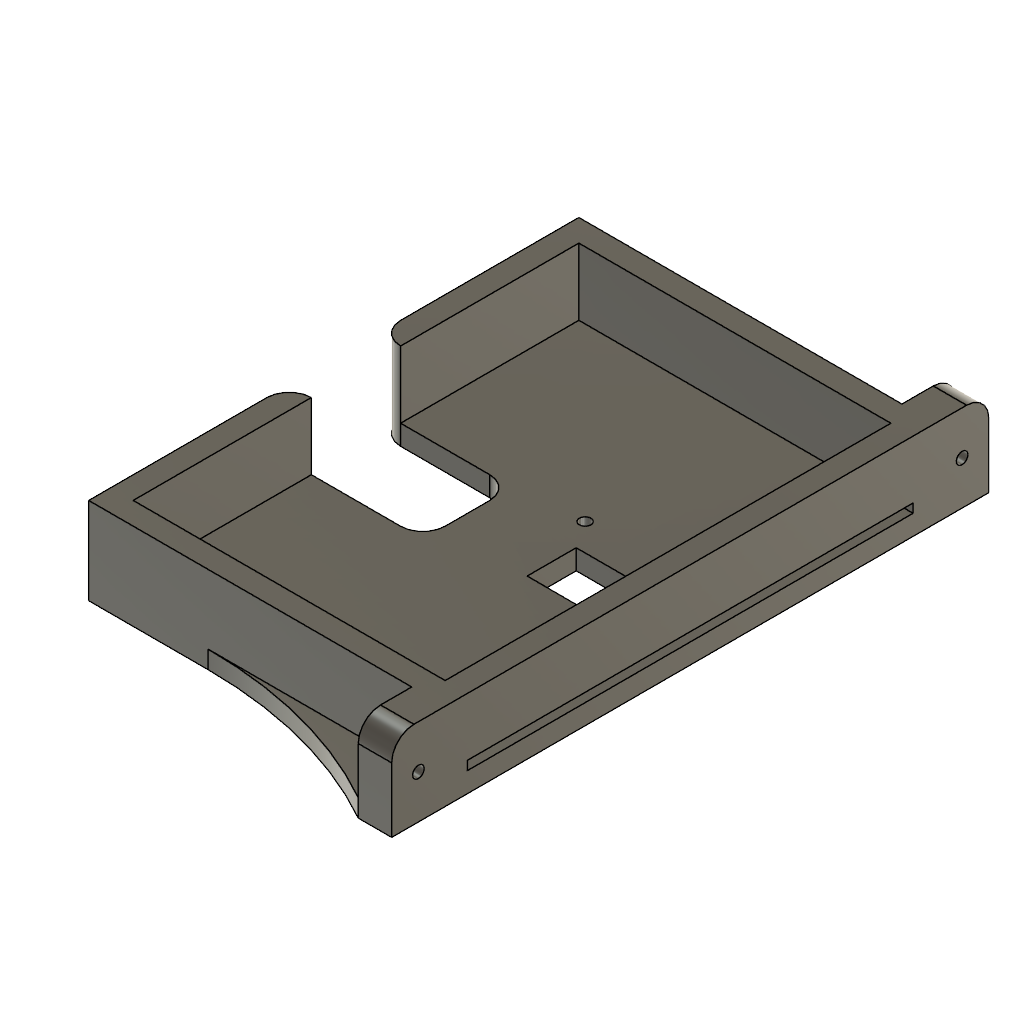
Upper_Card_Holder (Autodesk Fusion 360 design; units mm, degrees)
Autodesk Fusion 360 part; units mm, degrees
sketch "Çizim1" plane through (0, 0, 0) normal (0, 0, 1) x (1, 0, 0)
  line L0 (35, 50) -> (-35, 50)
  line L1 (-35, 50) -> (-35, -50)
  line L2 (-35, -50) -> (35, -50)
  line L3 (35, -50) -> (35, 50)
  line L4 (35, 50) -> (-35, -50) construction
  line L5 (-35, 50) -> (35, -50) construction
  line L6 (-40, -55) -> (40, -55)
  line L7 (40, -55) -> (40, 55)
  line L8 (40, 55) -> (-40, 55)
  line L9 (-40, 55) -> (-40, -55)
  dimension "d1" = 70
  dimension "d2" = 100
  dimension "d3" = 5
  constraint horizontal L0
  constraint perpendicular L0 L1
  constraint parallel L0 L2
  constraint parallel L1 L3
  constraint coincident L4 origin
  constraint coincident L5 origin
  measures "d1" distance of L1.end L2.end
  measures "d2" distance of L0.end L1.end
extrude "Ekstrüzyon1" add sketch "Çizim1" against normal blind 5 contours L0 L1 L2 L3 | L6 L7 L8 L9
extrude "Ekstrüzyon2" add sketch "Çizim1" along normal blind 20
sketch "Çizim2" plane through (0, -50, 0) normal (0, 1, 0) x (-1, 0, 0)
  line L0 (-35, 0) -> (35, 0)
  line L1 (35, 0) -> (35, 20)
  line L2 (35, 20) -> (-35, 20)
  line L3 (-35, 20) -> (-35, 0)
  line L4 (-35, 0) -> (35, 0)
  line L5 (35, 0) -> (35, 2.4)
  line L6 (35, 2.4) -> (-35, 2.4)
  line L7 (-35, 2.4) -> (-35, 0)
  dimension "d8" = 2.4
  constraint horizontal L4
  constraint vertical L5
  constraint horizontal L6
  constraint vertical L7
  constraint coincident L0.start L3.end
  measures "d8" distance of L0.start L6.end
sketch "Çizim3" plane through (0, 0, 20) normal (0, 0, 1) x (-1, 0, 0)
  line L0 (-35, -50) -> (-35, 50)
  line L1 (-35, 50) -> (35, 50)
  line L2 (35, 50) -> (35, -50)
  line L3 (35, -50) -> (-35, -50)
  line L4 (40, -55) -> (40, 55)
  line L5 (40, 55) -> (-40, 55)
  line L6 (-40, 55) -> (-40, -55)
  line L7 (-40, -55) -> (40, -55)
  line L8 (12, -12.5) -> (-12, -12.5)
  line L9 (-12, -12.5) -> (-12, -87.5)
  line L10 (-12, -87.5) -> (12, -87.5)
  line L11 (12, -87.5) -> (12, -12.5)
  line L12 (12, -12.5) -> (-12, -87.5) construction
  line L13 (-12, -12.5) -> (12, -87.5) construction
  point P0 (0, -50)
  dimension "d11" = 75
  constraint horizontal L8
  constraint perpendicular L8 L9
  constraint parallel L8 L10
  constraint parallel L9 L11
  constraint coincident L12 P0
  constraint coincident L13 P0
  constraint midpoint L3 P0
  measures "d11" distance of L8.end L9.end
sketch "Çizim4" plane through (0, 0, -5) normal (0, 0, -1) x (1, 0, 0)
  line L0 (40, -55) -> (40, 55)
  line L1 (40, 55) -> (-40, 55)
  line L2 (-40, 55) -> (-40, -55)
  line L3 (-40, -55) -> (40, -55)
  line L4 (14, -4.5) -> (24, -4.5)
  line L5 (24, -4.5) -> (24, 4.5)
  line L6 (24, 4.5) -> (14, 4.5)
  line L7 (14, 4.5) -> (14, -4.5)
  line L8 (14, -4.5) -> (24, 4.5) construction
  line L9 (24, -4.5) -> (14, 4.5) construction
  point P0 (19, 0)
  dimension "d19" = 10
  dimension "d20" = 9
  dimension "d75" = 16
  constraint horizontal L4
  constraint perpendicular L4 L5
  constraint parallel L4 L6
  constraint parallel L5 L7
  constraint midpoint L8 P0
  constraint horizontal origin P0
  measures "d19" distance of L5.end L6.end
  measures "d20" distance of L4.end L5.end
  measures "d75" distance of L0 L5
extrude "Ekstrüzyon5" cut sketch "Çizim4" against normal blind 5 contours L4 L5 L6 L7
sketch "Çizim5" plane through (0, 0, 0) normal (0, 0, 1) x (-1, 0, 0)
  line L0 (-14, -4.5) -> (-24, -4.5)
  line L1 (-24, -4.5) -> (-24, 4.5)
  line L2 (-24, 4.5) -> (-14, 4.5)
  line L3 (-14, 4.5) -> (-14, -4.5)
  line L4 (35, -50) -> (35, 50)
  line L5 (-35, 50) -> (-35, -50)
  line L6 (-35, -50) -> (35, -50)
  line L7 (-30.1, -0.5) -> (-28.6, -0.5)
  line L8 (-30.1, -0.5) -> (-30.1, -14.7)
  line L9 (-30.1, -0.5) -> (-30.1, 13.7)
  circle A0 centre (-30.1, 13.7) radius 1.3
  circle A1 centre (-30.1, -14.7) radius 1.3
  circle A2 centre (-30.1, -14.7) radius 3
  circle A3 centre (-30.1, 13.7) radius 3
  line L10 (35, 50) -> (-35, 50)
  line L11 (-33.2, -11.6) -> (-4.8, -11.6)
  line L12 (-4.8, -11.6) -> (-19, -11.6)
  circle A4 centre (-33.2, -11.6) radius 1.3
  circle A5 centre (-4.8, -11.6) radius 1.3
  point P0 (-19, -4.5)
  dimension "d23" = 14.2
  dimension "d24" = 14.2
  dimension "d25" = 2.6
  dimension "d26" = 2.6
  dimension "d27" = 6
  dimension "d28" = 6
  dimension "d43" = 9.2
  dimension "d44" = 16.1
  dimension "d59" = 16.1
  dimension "d60" = 28.4
  dimension "d61" = 2.6
  dimension "d62" = 2.6
  constraint perpendicular L0 L8
  constraint coincident L9.end A0.centre
  constraint coincident L8.end A1.centre
  constraint concentric A1 A2
  constraint concentric A0 A3
  constraint parallel L7 L11
  constraint midpoint L11 L12.end
  constraint coincident L11.start A4.centre
  constraint coincident L11.end L12.start
  constraint midpoint L0 P0
  constraint vertical L12.end P0
  measures "d23" distance of L7.start L8.end
  measures "d24" distance of L7.start L9.end
  measures "d25" diameter of A0
  measures "d26" diameter of A1
  measures "d27" diameter of A2
  measures "d28" diameter of A3
  measures "d43" distance of L2 L9.end
  measures "d44" distance of L3 L9.end
  measures "d59" distance of L2 L11
  measures "d60" distance of L11.start L11.end
  measures "d61" diameter of A4
  measures "d62" diameter of A5
extrude "Ekstrüzyon16" cut sketch "Çizim5" against normal blind 5 contours A4 | A5
sketch "Çizim7" plane through (40, 0, 0) normal (1, 0, 0) x (0, 1, 0)
  line L0 (-55, 20) -> (-55, -5)
  line L1 (-55, -5) -> (55, -5)
  line L2 (55, -5) -> (55, 20)
  line L3 (55, 20) -> (-55, 20)
  line L4 (-50, 1.5) -> (50, 1.5)
  line L5 (50, 1.5) -> (50, -0.5)
  line L6 (50, -0.5) -> (-50, -0.5)
  line L7 (-50, -0.5) -> (-50, 1.5)
  dimension "d52" = 2
  dimension "d53" = 5
  dimension "d54" = 5
  dimension "d55" = 4.5
  constraint horizontal L4
  constraint vertical L5
  constraint horizontal L6
  constraint vertical L7
  measures "d52" distance of L4 L6
  measures "d53" distance of L2 L5
  measures "d54" distance of L0 L7
  measures "d55" distance of L1 L6
extrude "Ekstrüzyon15" cut sketch "Çizim7" against normal blind 5 contours L4 L5 L6 L7
extrude "Ekstrüzyon17" cut 1 faces at (14, -1.5, -3.3333) along direction (-1, 0, 0) blind 5.1
extrude "Ekstrüzyon18" cut 1 faces at (24, 1.5, -3.3333) along direction (1, 0, 0) blind 5.1
extrude "Ekstrüzyon19" cut 1 faces at (15.6333, 4.5, -3.3333) along direction (0, 1, 0) blind 1
extrude "Ekstrüzyon20" cut 1 faces at (22.3667, -4.5, -3.3333) along direction (0, -1, 0) blind 1
extrude "Ekstrüzyon21" cut 1 faces at (-22.1593, 3.787, 0) along direction (0, 0, -1) blind 0.5
extrude "Ekstrüzyon22" cut 1 faces at (-38.3333, 16.6667, 20) along direction (0, 0, -1) blind 5.5
sketch "Çizim8" plane through (0, 0, -5) normal (0, 0, -1) x (1, 0, 0)
  line L0 (29.1, 5.5) -> (29.1, -5.5)
  line L1 (29.1, -5.5) -> (8.9, -5.5)
  line L2 (8.9, -5.5) -> (8.9, 5.5)
  line L3 (8.9, 5.5) -> (29.1, 5.5)
  circle A0 centre (4.8, -11.6) radius 1.3
  circle A1 centre (33.2, -11.6) radius 1.3
  line L4 (-40, 55) -> (-40, -55)
  line L5 (-40, -55) -> (40, -55)
  line L6 (40, -55) -> (40, 55)
  line L7 (40, 55) -> (-40, 55)
  line L8 (-40, -10) -> (-10, -10)
  line L9 (-10, -10) -> (-10, 10)
  line L10 (-10, 10) -> (-40, 10)
  line L11 (-40, 10) -> (-40, -10)
  constraint horizontal L8
  constraint vertical L9
  constraint horizontal L10
  constraint vertical L11
  constraint coincident L4 L8.start
extrude "Ekstrüzyon23" cut sketch "Çizim8" against normal blind 19.5 contours L4 L8 L9 L10 L11
fillet "Kavis2" radius 5 4 edges at (-10, 10, -2.75) (-10, -10, -2.75) (-40, 10, 4.75) (-40, -10, 4.75)
sketch "Çizim9" plane through (40, 0, 0) normal (1, 0, 0) x (0, 1, 0)
  line L0 (55, 14.5) -> (-55, 14.5)
  line L1 (-55, 14.5) -> (-55, -5)
  line L2 (-55, -5) -> (55, -5)
  line L3 (55, -5) -> (55, 14.5)
  line L4 (50, 1.5) -> (50, -0.5)
  line L5 (50, -0.5) -> (-50, -0.5)
  line L6 (-50, -0.5) -> (-50, 1.5)
  line L7 (-50, 1.5) -> (50, 1.5)
  line L8 (-55, 14.5) -> (-67, 14.5)
  line L9 (-67, 14.5) -> (-67, -5)
  line L10 (-67, -5) -> (-55, -5)
  line L11 (-55, -5) -> (-55, 14.5)
  circle A0 centre (-61, 4.75) radius 1.3
  dimension "d82" = 12
  dimension "d83" = 19.5
  dimension "d84" = 2.6
  dimension "d85" = 6
  dimension "d86" = 9.75
  constraint horizontal L8
  constraint vertical L9
  constraint horizontal L10
  constraint vertical L11
  constraint coincident L0.end L1.start
  measures "d82" distance of L0.end L8.end
  measures "d83" distance of L8.end L9.end
  measures "d84" diameter of A0
  measures "d85" distance of L11 A0.centre
  measures "d86" distance of L10 A0.centre
extrude "Ekstrüzyon24" add sketch "Çizim9" against normal blind 7.5 contours L1 L8 L9 L10 L11
sketch "Çizim10" plane through (0, 0, -5) normal (0, 0, -1) x (1, 0, 0)
  arc A0 (-40, 15) -> (-35, 10) centre (-35, 15) ccw
  line L0 (-35, 10) -> (-15, 10)
  arc A1 (-10, 5) -> (-15, 10) centre (-15, 5) ccw
  line L1 (-10, 5) -> (-10, -5)
  arc A2 (-15, -10) -> (-10, -5) centre (-15, -5) ccw
  line L2 (-15, -10) -> (-35, -10)
  arc A3 (-35, -10) -> (-40, -15) centre (-35, -15) ccw
  line L3 (-40, -15) -> (-40, -55)
  line L4 (-40, -55) -> (40, -55)
  line L5 (40, -55) -> (40, 67)
  line L6 (40, 67) -> (32.5, 67)
  line L7 (32.5, 67) -> (32.5, 55)
  line L8 (32.5, 55) -> (-40, 55)
  line L9 (-40, 55) -> (-40, 15)
  line L10 (29.1, 5.5) -> (29.1, -5.5)
  line L11 (29.1, -5.5) -> (8.9, -5.5)
  line L12 (8.9, -5.5) -> (8.9, 5.5)
  line L13 (8.9, 5.5) -> (29.1, 5.5)
  circle A4 centre (4.8, -11.6) radius 1.3
  circle A5 centre (33.2, -11.6) radius 1.3
  line L14 (32.5, 67) -> (11.7154, 55)
  line L15 (32.5, 67) -> (56.5, 67) construction
  dimension "d89" = 150
  constraint horizontal L15
  constraint coincident L6.end L7.start
  constraint coincident L8 L14.end
  measures "d89" angle of L14 L15
extrude "Ekstrüzyon25" add sketch "Çizim10" against normal blind 4 contours L7 L8 L14
fillet "Kavis3" radius 93 1 edges at (11.7154, -55, -3)
mirror "Ayna1" about plane through (0, 0, 0) normal (0, 1, 0) of "Ekstrüzyon24", "Ekstrüzyon25"
fillet "Kavis4" radius 93 1 edges at (11.7154, 55, -3)
fillet "Kavis5" radius 5 2 edges at (36.25, 67, 14.5) (36.25, -67, 14.5)
equation "d23 = 6 mm + 13.20 mm - 5 mm"
equation "d24 = 6 mm + 13.20 mm - 5 mm"
equation "d44 = 9 mm + 7.1 mm"
equation "d86 = ( 19.5 / 2 ) * 1 mm"
